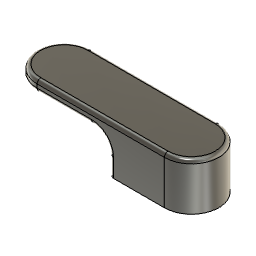
BambuHandle (Autodesk Fusion 360 design; units mm, degrees)
Autodesk Fusion 360 part; units mm, degrees
note: some values were not read from the file. Set by a fixed rule: which sketch regions a step uses.
sketch "Sketch1" plane through (0, 0, 0) normal (0, 0, 1) x (1, 0, 0)
  line L0 (0, 0) -> (15, 0)
  line L1 (15, 0) -> (15, 15)
  line L2 (15, 15) -> (0, 15)
  line L3 (0, 15) -> (0, 0)
  circle A0 centre (15, 7.5) radius 7.5
  circle A1 centre (15, 7.5) radius 0.85
  circle A2 centre (5, 7.5) radius 0.85
  dimension "d1" = 15
  dimension "d2" = 15
  dimension "d3" = 1.7
  dimension "d4" = 10
  dimension "d5" = 7.5
  dimension "d6" = 1.7
  constraint horizontal L0
  constraint vertical L1
  constraint horizontal L2
  constraint vertical L3
  constraint coincident L0.start L3.end
  constraint midpoint L1 A0.centre
  constraint coincident L1.end A0
  constraint concentric A0 A1
  measures "d1" distance of L0.start L2.end
  measures "d2" distance of L0.start L0.end
  measures "d3" diameter of A1
  measures "d4" horizontal distance of A0.centre A2.centre
  measures "d5" distance of L0 A2.centre
  measures "d6" diameter of A2
extrude "Extrude1" add sketch "Sketch1" along normal blind 10 contours L0 L2 L3 A0 | L1 A0 A1 | L1 A0 A1
sketch "Sketch2" plane through (0, 0, 10) normal (0, 0, 1) x (-1, 0, 0)
  circle A0 centre (-5, -7.5) radius 0.85
  circle A1 centre (-15, -7.5) radius 0.85
  arc A2 (-15, 0) -> (-15, -15) centre (-15, -7.5) ccw
  line L0 (-15, -15) -> (0, -15)
  line L1 (0, -15) -> (0, 0)
  line L2 (0, 0) -> (-15, 0)
  line L3 (0, -15) -> (-15, -15)
  arc A3 (-15, 0) -> (-15, -15) centre (-15, -7.5) ccw
  line L4 (0, 0) -> (-15, 0)
  line L5 (0, -15) -> (0, 0)
  line L6 (0, 0) -> (20, 0)
  line L7 (20, 0) -> (20, -15)
  line L8 (20, -15) -> (0, -15)
  line L9 (0, -15) -> (0, 0)
  arc A4 (20, -15) -> (20, 0) centre (20, -7.5) ccw
  dimension "d9" = 20
  dimension "d10" = 15
  constraint coincident L0.end L1.start
  constraint coincident A2.end L0.start
  constraint coincident A2.start L2.end
  constraint tangent L3 A3
  constraint coincident L1.end L2.start
  constraint horizontal L6
  constraint vertical L7
  constraint horizontal L8
  constraint vertical L9
  constraint tangent L8 A4
  measures "d9" distance of L7.end L0.end
  measures "d10" distance of L6 L8
extrude "Extrude2" add sketch "Sketch2" along normal blind 3 contours A0 | A1 | A2 L0 L1 L2 L3 A3 L4 L5 L9 | L1 L5 L6 L7 L8 L9 | L7 A4
fillet "Fillet1" radius 1 1 faces at (-1.6667, 5, 13)
fillet "Fillet2" radius 5 1 edges at (0, 7.5, 10)
fillet "Fillet3" radius 1 7 edges at (0, 15, 2.5) (-1.4645, 15, 8.5355) (-12.5, 15, 10) (-27.5, 7.5, 10) (-12.5, 0, 10) (-1.4645, 0, 8.5355) (0, 0, 2.5)
sketch "Sketch3" plane through (0, 0, 0) normal (0, 0, -1) x (1, 0, 0)
  arc A0 (1, 0) -> (0, -1) centre (1, -1) ccw
  line L0 (0, -1) -> (0, -14)
  arc A1 (0, -14) -> (1, -15) centre (1, -14) ccw
  line L1 (1, -15) -> (15, -15)
  arc A2 (15, -15) -> (15, 0) centre (15, -7.5) ccw
  line L2 (15, 0) -> (1, 0)
  line L3 (2, -2) -> (2, -13)
  line L4 (2, -13) -> (15, -13)
  arc A3 (15, -13) -> (15, -2) centre (15, -7.5) ccw
  line L5 (15, -2) -> (2, -2)
  circle A4 centre (5, -7.5) radius 0.85
  circle A5 centre (15, -7.5) radius 0.85
  dimension "d21" = -2
extrude "Extrude3" cut sketch "Sketch3" along normal blind 0 and the other way blind 3.15 contours L3 L4 A3 L5
fillet "Fillet4" radius 2 2 edges at (2, 13, 1.575) (2, 2, 1.575)
fillet "Fillet5" radius 1 6 edges at (2.5858, 12.4142, 3.15) (2, 7.5, 3.15) (2.5858, 2.5858, 3.15) (9.5, 2, 3.15) (20.5, 7.5, 3.15) (9.5, 13, 3.15)
fillet "Fillet6" radius 1 6 edges at (2.5858, 12.4142, 0) (2, 7.5, 0) (2.5858, 2.5858, 0) (9.5, 2, 0) (20.5, 7.5, 0) (9.5, 13, 0)
chamfer "Chamfer2" distance 0.3 angle 45 2 edges at (14.2075, 7.8074, 3.15) (4.2075, 7.8074, 3.15)
